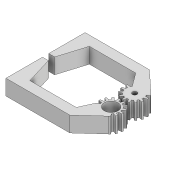
# Autodesk Inventor part: dientes mas afilados
Saved by Autodesk Inventor 2021 (Build 250183000, 183)
## iProperties
Created: 2022-06-07
Part Number: dientes mas afilados
Material: Genérico
Document SubType Name: Modeling
Designer: orgyn
Density: 1 g/cm^3
Appearance: Valor por defecto
Author: orgyn
Autodesk Inventor part; units mm, degrees
ref_plane "YZ Plane" through (0, 0, 0) normal (1, 0, 0) x (0, 1, 0)
ref_plane "XZ Plane" through (0, 0, 0) normal (0, 1, 0) x (-1, 0, 0)
ref_plane "XY Plane" through (0, 0, 0) normal (0, 0, 1) x (1, 0, 0)
sketch "Boceto1" plane through (0, 0, 0) normal (0, 1, 0) x (-1, 0, 0)
  circle A0 centre (0, 0) radius 4.5
  line L0 (7.4833, 0.4997) -> (5.4489, 0.7483)
  line L1 (7.4833, -0.4997) -> (5.4489, -0.7483)
  line L2 (6.5254, 3.6971) -> (4.5846, 3.0383)
  line L3 (6.9591, 2.7967) -> (5.2339, 1.69)
  line L4 (4.2751, 6.1623) -> (2.8123, 4.7266)
  line L5 (5.0565, 5.5391) -> (3.9823, 3.7936)
  line L6 (1.178, 7.4069) -> (0.483, 5.4788)
  line L7 (2.1524, 7.1845) -> (1.942, 5.1457)
  line L8 (-2.1524, 7.1845) -> (-1.942, 5.1457)
  line L9 (-1.178, 7.4069) -> (-0.483, 5.4788)
  line L10 (-5.0565, 5.5391) -> (-3.9823, 3.7936)
  line L11 (-4.2751, 6.1623) -> (-2.8123, 4.7266)
  line L12 (-6.9591, 2.7967) -> (-5.2339, 1.69)
  line L13 (-6.5254, 3.6971) -> (-4.5846, 3.0383)
  line L14 (-7.4833, -0.4997) -> (-5.4489, -0.7483)
  line L15 (-7.4833, 0.4997) -> (-5.4489, 0.7483)
  line L16 (-6.5254, -3.6971) -> (-4.5846, -3.0383)
  line L17 (-6.9591, -2.7967) -> (-5.2339, -1.69)
  line L18 (-4.2751, -6.1623) -> (-2.8123, -4.7266)
  line L19 (-5.0565, -5.5391) -> (-3.9823, -3.7936)
  line L20 (-1.178, -7.4069) -> (-0.483, -5.4788)
  line L21 (-2.1524, -7.1845) -> (-1.942, -5.1457)
  line L22 (2.1524, -7.1845) -> (1.942, -5.1457)
  line L23 (1.178, -7.4069) -> (0.483, -5.4788)
  line L24 (5.0565, -5.5391) -> (3.9823, -3.7936)
  line L25 (4.2751, -6.1623) -> (2.8123, -4.7266)
  line L26 (6.9591, -2.7967) -> (5.2339, -1.69)
  line L27 (6.5254, -3.6971) -> (4.5846, -3.0383)
  arc A1 (5.0565, 5.5391) -> (4.2751, 6.1623) centre (0, 0) ccw
  arc A2 (2.1524, 7.1845) -> (1.178, 7.4069) centre (0, 0) ccw
  arc A3 (-1.178, 7.4069) -> (-2.1524, 7.1845) centre (0, 0) ccw
  arc A4 (-4.2751, 6.1623) -> (-5.0565, 5.5391) centre (0, 0) ccw
  arc A5 (-6.5254, 3.6971) -> (-6.9591, 2.7967) centre (0, 0) ccw
  arc A6 (-7.4833, 0.4997) -> (-7.4833, -0.4997) centre (0, 0) ccw
  arc A7 (-6.9591, -2.7967) -> (-6.5254, -3.6971) centre (0, 0) ccw
  arc A8 (-5.0565, -5.5391) -> (-4.2751, -6.1623) centre (0, 0) ccw
  arc A9 (-2.1524, -7.1845) -> (-1.178, -7.4069) centre (0, 0) ccw
  arc A10 (1.178, -7.4069) -> (2.1524, -7.1845) centre (0, 0) ccw
  arc A11 (4.2751, -6.1623) -> (5.0565, -5.5391) centre (0, 0) ccw
  arc A12 (6.5254, -3.6971) -> (6.9591, -2.7967) centre (0, 0) ccw
  arc A13 (7.4833, -0.4997) -> (7.4833, 0.4997) centre (0, 0) ccw
  arc A14 (6.9591, 2.7967) -> (6.5254, 3.6971) centre (0, 0) ccw
  arc A15 (5.4489, 0.7483) -> (5.2339, 1.69) centre (0, 0) ccw
  arc A16 (4.5846, 3.0383) -> (3.9823, 3.7936) centre (0, 0) ccw
  arc A17 (5.2339, -1.69) -> (5.358, -1.2419) centre (0, 0) ccw
  arc A18 (5.358, 1.2419) -> (5.2339, 1.69) centre (0, 0) ccw
  arc A19 (4.5846, 3.0383) -> (3.9823, 3.7936) centre (0, 0) ccw
  arc A20 (2.8123, 4.7266) -> (1.942, 5.1457) centre (0, 0) ccw
  arc A21 (2.8123, 4.7266) -> (1.942, 5.1457) centre (0, 0) ccw
  arc A22 (0.483, 5.4788) -> (-0.483, 5.4788) centre (0, 0) ccw
  arc A23 (0.483, 5.4788) -> (-0.483, 5.4788) centre (0, 0) ccw
  arc A24 (-1.942, 5.1457) -> (-2.8123, 4.7266) centre (0, 0) ccw
  arc A25 (-1.942, 5.1457) -> (-2.8123, 4.7266) centre (0, 0) ccw
  arc A26 (-3.9823, 3.7936) -> (-4.5846, 3.0383) centre (0, 0) ccw
  arc A27 (-3.9823, 3.7936) -> (-4.5846, 3.0383) centre (0, 0) ccw
  arc A28 (-5.2339, 1.69) -> (-5.4489, 0.7483) centre (0, 0) ccw
  arc A29 (-5.2339, 1.69) -> (-5.4489, 0.7483) centre (0, 0) ccw
  arc A30 (-5.4489, -0.7483) -> (-5.2339, -1.69) centre (0, 0) ccw
  arc A31 (-5.4489, -0.7483) -> (-5.2339, -1.69) centre (0, 0) ccw
  arc A32 (-4.5846, -3.0383) -> (-3.9823, -3.7936) centre (0, 0) ccw
  arc A33 (-4.5846, -3.0383) -> (-3.9823, -3.7936) centre (0, 0) ccw
  arc A34 (-2.8123, -4.7266) -> (-1.942, -5.1457) centre (0, 0) ccw
  arc A35 (-2.8123, -4.7266) -> (-1.942, -5.1457) centre (0, 0) ccw
  arc A36 (-0.483, -5.4788) -> (0.483, -5.4788) centre (0, 0) ccw
  arc A37 (-0.483, -5.4788) -> (0.483, -5.4788) centre (0, 0) ccw
  arc A38 (1.942, -5.1457) -> (2.8123, -4.7266) centre (0, 0) ccw
  arc A39 (1.942, -5.1457) -> (2.8123, -4.7266) centre (0, 0) ccw
  arc A40 (3.9823, -3.7936) -> (4.5846, -3.0383) centre (0, 0) ccw
  arc A41 (3.9823, -3.7936) -> (4.5846, -3.0383) centre (0, 0) ccw
  arc A42 (5.2339, -1.69) -> (5.4489, -0.7483) centre (0, 0) ccw
  line L28 (0, 0) -> (0, 10.0549)
  line L29 (8.723, 17.9975) -> (50, 17.9975)
  line L30 (40.9223, 11.63) -> (10.9223, 11.63)
  line L31 (10.9223, 11.63) -> (4.3001, 3.4292)
  arc A43 (7.4564, -14.3927) -> (7.2829, -13.4084) centre (0, -15.2) ccw
  arc A44 (6.3677, -11.2374) -> (5.7843, -10.4259) centre (0, -15.2) ccw
  line L32 (5.7843, -10.4259) -> (3.9874, -11.4117)
  line L33 (6.3677, -11.2374) -> (4.8609, -12.6268)
  line L34 (7.2829, -13.4084) -> (5.2362, -13.5169)
  circle A45 centre (0, -15.2) radius 4.5
  arc A46 (4.0178, -8.867) -> (3.1401, -8.389) centre (0, -15.2) ccw
  arc A47 (5.0609, -13.0466) -> (4.8609, -12.6268) centre (0, -15.2) ccw
  arc A48 (5.2362, -13.5169) -> (4.8609, -12.6268) centre (0, -15.2) ccw
  arc A49 (3.9874, -11.4117) -> (3.2631, -10.7725) centre (0, -15.2) ccw
  arc A50 (3.9874, -11.4117) -> (3.2631, -10.7725) centre (0, -15.2) ccw
  line L35 (4.0178, -8.867) -> (3.2631, -10.7725)
  line L36 (3.1401, -8.389) -> (1.9488, -10.0568)
  arc A51 (1.9488, -10.0568) -> (1.0189, -9.7952) centre (0, -15.2) ccw
  arc A52 (1.9488, -10.0568) -> (1.0189, -9.7952) centre (0, -15.2) ccw
  line L37 (0.8721, -7.7509) -> (1.0189, -9.7952)
  line L38 (-0.1261, -7.7011) -> (-0.4757, -9.7206)
  arc A53 (-0.4757, -9.7206) -> (-1.427, -9.8884) centre (0, -15.2) ccw
  arc A54 (-0.4757, -9.7206) -> (-1.427, -9.8884) centre (0, -15.2) ccw
  arc A55 (0.8721, -7.7509) -> (-0.1261, -7.7011) centre (0, -15.2) ccw
  arc A56 (4.5806, -18.2444) -> (5.0426, -17.3961) centre (0, -15.2) ccw
  arc A57 (4.5806, -18.2444) -> (5.0426, -17.3961) centre (0, -15.2) ccw
  arc A58 (5.2802, -20.5263) -> (5.9415, -19.7769) centre (0, -15.2) ccw
  arc A59 (7.0683, -17.7078) -> (7.339, -16.7457) centre (0, -15.2) ccw
  line L39 (5.2802, -20.5263) -> (3.5903, -19.3665)
  line L40 (5.9415, -19.7769) -> (4.5806, -18.2444)
  arc A60 (5.4479, -15.9555) -> (5.4922, -15.4926) centre (0, -15.2) ccw
  arc A61 (5.4479, -15.9555) -> (5.496, -14.9907) centre (0, -15.2) ccw
  line L41 (7.339, -16.7457) -> (5.4479, -15.9555)
  line L42 (7.0683, -17.7078) -> (5.0426, -17.3961)
  line L43 (7.4564, -14.3927) -> (5.496, -14.9907)
  line L44 (-7.0683, -12.6922) -> (-5.0426, -13.0039)
  arc A62 (-4.5806, -12.1556) -> (-5.0426, -13.0039) centre (0, -15.2) ccw
  arc A63 (-4.5806, -12.1556) -> (-5.0426, -13.0039) centre (0, -15.2) ccw
  line L45 (-5.9415, -10.6231) -> (-4.5806, -12.1556)
  arc A64 (-2.806, -10.4696) -> (-3.5903, -11.0335) centre (0, -15.2) ccw
  arc A65 (-2.806, -10.4696) -> (-3.5903, -11.0335) centre (0, -15.2) ccw
  line L46 (-5.2802, -9.8737) -> (-3.5903, -11.0335)
  arc A66 (-5.2802, -9.8737) -> (-5.9415, -10.6231) centre (0, -15.2) ccw
  arc A67 (-5.4479, -14.4445) -> (-5.496, -15.4093) centre (0, -15.2) ccw
  arc A68 (-5.4479, -14.4445) -> (-5.496, -15.4093) centre (0, -15.2) ccw
  arc A69 (-7.0683, -12.6922) -> (-7.339, -13.6543) centre (0, -15.2) ccw
  line L47 (-7.339, -13.6543) -> (-5.4479, -14.4445)
  arc A70 (-5.2362, -16.8831) -> (-4.8609, -17.7732) centre (0, -15.2) ccw
  arc A71 (-5.2362, -16.8831) -> (-4.8609, -17.7732) centre (0, -15.2) ccw
  line L48 (-7.4564, -16.0073) -> (-5.496, -15.4093)
  line L49 (-7.2829, -16.9916) -> (-5.2362, -16.8831)
  line L50 (-6.3677, -19.1626) -> (-4.8609, -17.7732)
  line L51 (-5.7843, -19.9741) -> (-3.9874, -18.9883)
  arc A72 (-6.3677, -19.1626) -> (-5.7843, -19.9741) centre (0, -15.2) ccw
  line L52 (-4.0178, -21.533) -> (-3.2631, -19.6275)
  arc A73 (-4.0178, -21.533) -> (-3.1401, -22.011) centre (0, -15.2) ccw
  arc A74 (-1.9488, -20.3432) -> (-1.0189, -20.6048) centre (0, -15.2) ccw
  arc A75 (-1.9488, -20.3432) -> (-1.0189, -20.6048) centre (0, -15.2) ccw
  arc A76 (0.4757, -20.6794) -> (1.427, -20.5116) centre (0, -15.2) ccw
  arc A77 (0.4757, -20.6794) -> (1.427, -20.5116) centre (0, -15.2) ccw
  line L53 (2.4463, -22.2898) -> (1.427, -20.5116)
  line L54 (-3.1401, -22.011) -> (-1.9488, -20.3432)
  arc A78 (-2.4463, -8.1102) -> (-3.3673, -8.4984) centre (0, -15.2) ccw
  line L55 (-2.4463, -8.1102) -> (-1.427, -9.8884)
  line L56 (-3.3673, -8.4984) -> (-2.806, -10.4696)
  arc A79 (2.806, -19.9304) -> (3.5903, -19.3665) centre (0, -15.2) ccw
  arc A80 (2.4463, -22.2898) -> (3.3673, -21.9016) centre (0, -15.2) ccw
  line L57 (3.3673, -21.9016) -> (2.806, -19.9304)
  arc A81 (2.806, -19.9304) -> (3.5903, -19.3665) centre (0, -15.2) ccw
  line L58 (0.1261, -22.6989) -> (0.4757, -20.6794)
  arc A82 (-0.8721, -22.6491) -> (0.1261, -22.6989) centre (0, -15.2) ccw
  line L59 (-0.8721, -22.6491) -> (-1.0189, -20.6048)
  arc A83 (-3.9874, -18.9883) -> (-3.2631, -19.6275) centre (0, -15.2) ccw
  arc A84 (-3.9874, -18.9883) -> (-3.2631, -19.6275) centre (0, -15.2) ccw
  line L60 (40.9223, -26.83) -> (10.9223, -26.83)
  line L61 (50, -33.13) -> (50, -4.6936)
  line L62 (-7.4564, -16.0073) -> (-7.2829, -16.9916)
  line L63 (46.202, -5.6) -> (50, -5.6)
  line L64 (46.202, -9.6) -> (50, -9.6)
  line L65 (40.9223, 11.63) -> (46.202, -5.6)
  line L66 (46.202, -9.6) -> (40.9223, -26.83)
  line L67 (8.723, 17.9975) -> (-4.2751, 6.1623)
  line L68 (50, -5.6) -> (50, 17.9975)
  line L69 (10.9223, -33.13) -> (40.9223, -33.13)
  line L70 (40.9223, -33.13) -> (50, -33.13)
  line L71 (10.9223, -33.13) -> (8.4098, -33.13)
  line L72 (10.9223, -26.83) -> (4.5806, -18.2444)
  line L73 (8.4098, -33.13) -> (-5.7843, -19.9741)
  line L74 (10.9223, 11.63) -> (6.9591, 2.7967)
  circle A85 centre (0, -15.2) radius 1.5
  point P0 (5.4922, -15.4926)
  point P1 (5.0609, -13.0466)
  point P2 (5.358, -1.2419)
  dimension "d1" = 9
  dimension "d11" = 360
  dimension "d16" = 20
  dimension "d19" = 30
  dimension "d30" = 6.3
  dimension "d31" = 3
  constraints: 167 point on circle, 150 end point, 86 centre point, 7 coincident, 5 point on line, 3 perpendicular, 1 horizontal, 1 vertical, 85 other
  measures "d1" diameter of A0
  measures "d16" distance of L28.start L29.start
  measures "d19" distance of L30.start L30.end
  measures "d30" distance of L60.end L69.start
  measures "d31" diameter of A85
extrude "Extrusión1" add sketch "Boceto1" along normal blind 10 contours A13 L1 A42 A17 L26 A12 L27 A40 L24 A11 L25 A38 L22 A10 L23 A36 L20 A9 L21 A34 L18 A8 L19 A32 L16 A7 L17 A30 L14 A6 L15 A28 L12 A5 L13 A26 L10 A4 L11 A24 L8 A3 L9 A22 L6 A2 L7 A20 L4 A1 L5 A16 L2 A14 L3 A15 L0 | A14 L2 A16 L31 L74 | L31 A16 L5 A1 L4 A20 L7 A2 L6 A22 L28 L67 L29 L68 L61 L63 L65 L30 | L28 A22 L9 A3 L8 A24 L11 L67 | L43 A61 A60 L41 A59 L42 A56 L72 A58 L39 A79 L57 A80 L53 A76 L58 A82 L59 A74 L54 A73 L52 A83 L51 A72 L50 A70 L49 L62 L48 A67 L47 A69 L44 A62 L45 A66 L46 A64 L56 A78 L55 A53 L38 A55 L37 A51 L36 A46 L35 A49 L32 A44 L33 A47 A48 L34 A43 | L72 L60 L66 L64 L61 L70 L69 L71 L73 L51 A83 L52 A73 L54 A74 L59 A82 L58 A76 L53 A80 L57 A79 L39 A58 | A45
